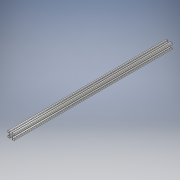
# Autodesk Inventor part: Aluminium Profile 2020 500mm
Saved by Autodesk Inventor 2019 (Build 230136000, 136)
## iProperties
Created: 2020-11-22
Part Number: Aluminium Profile 2020 500mm
Material: Aluminum 6061
Document SubType Name: Modeling
Designer: asus
Density: 2.7 g/cm^3
Appearance: Aluminum - Polished
Author: asus
Autodesk Inventor part; units mm, degrees
ref_plane "YZ Plane" through (0, 0, 0) normal (1, 0, 0) x (0, 1, 0)
ref_plane "XZ Plane" through (0, 0, 0) normal (0, 1, 0) x (-1, 0, 0)
ref_plane "XY Plane" through (0, 0, 0) normal (0, 0, 1) x (1, 0, 0)
sketch "Sketch1" plane through (0, 0, 0) normal (0, 0, 1) x (1, 0, 0)
  line L0 (-33.69, 10) -> (-33.9, 10.21)
  line L1 (-33.9, 10.21) -> (-33.9, 12.8393)
  line L2 (-33.9, 12.8393) -> (-36.5607, 15.5)
  line L3 (-36.5607, 15.5) -> (-38.2, 15.5)
  line L4 (-38.2, 15.5) -> (-38.2, 13.395)
  line L5 (-38.2, 13.395) -> (-38.815, 13.395)
  line L6 (-38.815, 13.395) -> (-40, 14.58)
  line L7 (-40, 14.58) -> (-40, 18.5)
  arc A0 (-38.5, 20) -> (-40, 18.5) centre (-38.5, 18.5) ccw
  line L8 (-38.5, 20) -> (-34.58, 20)
  line L9 (-34.58, 20) -> (-33.395, 18.815)
  line L10 (-33.395, 18.815) -> (-33.395, 18.2)
  line L11 (-33.395, 18.2) -> (-35.5, 18.2)
  line L12 (-35.5, 18.2) -> (-35.5, 16.5607)
  line L13 (-35.5, 16.5607) -> (-32.8393, 13.9)
  line L14 (-32.8393, 13.9) -> (-30.21, 13.9)
  line L15 (-30.21, 13.9) -> (-30, 13.69)
  circle A1 centre (-30, 10) radius 2.3
  line L16 (-30.21, 6.1) -> (-30, 6.31)
  line L17 (-32.8393, 6.1) -> (-30.21, 6.1)
  line L18 (-33.9, 9.79) -> (-33.9, 7.1607)
  line L19 (-33.69, 10) -> (-33.9, 9.79)
  line L20 (-33.395, 1.185) -> (-33.395, 1.8)
  line L21 (-35.5, 3.4393) -> (-32.8393, 6.1)
  line L22 (-33.395, 1.8) -> (-35.5, 1.8)
  line L23 (-35.5, 1.8) -> (-35.5, 3.4393)
  line L24 (-34.58, 0) -> (-33.395, 1.185)
  line L25 (-33.9, 7.1607) -> (-36.5607, 4.5)
  line L26 (-36.5607, 4.5) -> (-38.2, 4.5)
  line L27 (-38.2, 4.5) -> (-38.2, 6.605)
  line L28 (-38.2, 6.605) -> (-38.815, 6.605)
  line L29 (-38.815, 6.605) -> (-40, 5.42)
  line L30 (-38.5, 0) -> (-34.58, 0)
  arc A2 (-40, 1.5) -> (-38.5, 0) centre (-38.5, 1.5) ccw
  line L31 (-40, 5.42) -> (-40, 1.5)
  line L32 (-29.79, 13.9) -> (-30, 13.69)
  line L33 (-27.1607, 13.9) -> (-29.79, 13.9)
  line L34 (-26.1, 10.21) -> (-26.1, 12.8393)
  line L35 (-26.31, 10) -> (-26.1, 10.21)
  line L36 (-26.605, 18.815) -> (-26.605, 18.2)
  line L37 (-24.5, 16.5607) -> (-27.1607, 13.9)
  line L38 (-26.605, 18.2) -> (-24.5, 18.2)
  line L39 (-24.5, 18.2) -> (-24.5, 16.5607)
  line L40 (-25.42, 20) -> (-26.605, 18.815)
  line L41 (-26.1, 12.8393) -> (-23.4393, 15.5)
  line L42 (-23.4393, 15.5) -> (-21.8, 15.5)
  line L43 (-21.8, 15.5) -> (-21.8, 13.395)
  line L44 (-21.8, 13.395) -> (-21.185, 13.395)
  line L45 (-21.185, 13.395) -> (-20, 14.58)
  line L46 (-21.5, 20) -> (-25.42, 20)
  arc A3 (-20, 18.5) -> (-21.5, 20) centre (-21.5, 18.5) ccw
  line L47 (-20, 14.58) -> (-20, 18.5)
  line L48 (-29.79, 6.1) -> (-30, 6.31)
  line L49 (-26.605, 1.185) -> (-26.605, 1.8)
  line L50 (-27.1607, 6.1) -> (-29.79, 6.1)
  line L51 (-26.1, 9.79) -> (-26.1, 7.1607)
  line L52 (-26.31, 10) -> (-26.1, 9.79)
  line L53 (-24.5, 3.4393) -> (-27.1607, 6.1)
  line L54 (-26.605, 1.8) -> (-24.5, 1.8)
  line L55 (-24.5, 1.8) -> (-24.5, 3.4393)
  line L56 (-25.42, 0) -> (-26.605, 1.185)
  line L57 (-26.1, 7.1607) -> (-23.4393, 4.5)
  line L58 (-23.4393, 4.5) -> (-21.8, 4.5)
  line L59 (-21.8, 4.5) -> (-21.8, 6.605)
  line L60 (-21.8, 6.605) -> (-21.185, 6.605)
  line L61 (-21.5, 0) -> (-25.42, 0)
  line L62 (-21.185, 6.605) -> (-20, 5.42)
  line L63 (-20, 5.42) -> (-20, 1.5)
  arc A4 (-21.5, 0) -> (-20, 1.5) centre (-21.5, 1.5) ccw
  constraints: 128 end point, 8 point on circle, 5 centre point
extrude "Extrusion6" add sketch "Sketch1" along normal blind 500
body "Solid6"
